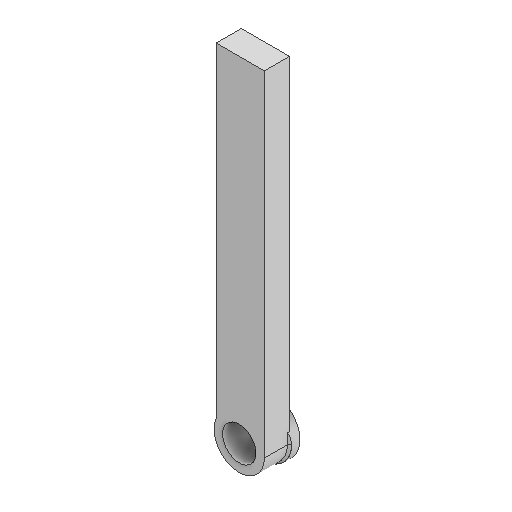
# Autodesk Inventor part: slide_clips_4mm
Saved by Autodesk Inventor 2023 (Build 270158000, 158)
## iProperties
Created: 2021-07-20
Part Number: slide_clips_4mm
Material: Generic
Document SubType Name: Modeling
Designer: CDT
Density: 1 g/cm^3
Appearance: Default
Author: CDT
Autodesk Inventor part; units mm, degrees
ref_plane "YZ Plane" through (0, 0, 0) normal (1, 0, 0) x (0, 1, 0)
ref_plane "XZ Plane" through (0, 0, 0) normal (0, 1, 0) x (-1, 0, 0)
ref_plane "XY Plane" through (0, 0, 0) normal (0, 0, 1) x (1, 0, 0)
sketch "Sketch1" plane through (0, 0, 0) normal (0, 0, 1) x (1, 0, 0)
  circle A0 centre (-24.0055, -25.7521) radius 3.25
  circle A1 centre (-24.0055, -25.7521) radius 2
  point P0 (0, 0)
  dimension "d0" = 6.5
  dimension "d1" = 4
  constraints: 2 centre point, 1 coincident
  measures "d0" diameter of A0
  measures "d1" diameter of A1
extrude "Extrusion1" add sketch "Sketch1" along normal blind 1
sketch "Sketch2" plane through (-24.0055, -25.7521, 1) normal (0, 0, 1) x (1, 0, 0)
  circle A0 centre (0, 0) radius 3
  circle A1 centre (0, 0) radius 2
  line L0 (0, 0) -> (-2.75, 0)
  line L1 (-2.75, 0) -> (-2.75, 40)
  line L2 (-2.75, 40) -> (0, 40)
  line L3 (0, 40) -> (0, 0)
  line L4 (0, 0) -> (3, 0)
  line L5 (3, 0) -> (3, 40)
  line L6 (3, 40) -> (0, 40)
  line L7 (0, 40) -> (0, 0)
  point P0 (24.0055, 25.7521)
  point P1 (-2.75, 1.199)
  point P2 (3, 0)
  point P3 (0, 40)
  dimension "d4" = 40
  dimension "d5" = 3
  dimension "d8" = 4
  dimension "d9" = 6
  constraints: 16 end point, 4 parallel, 2 centre point, 2 horizontal, 2 perpendicular, 1 coincident, 1 point on line
  measures "d4" distance of L0.end L1.end
  measures "d5" distance of L6.end L5.end
  measures "d8" diameter of A1
  measures "d9" diameter of A0
extrude "Extrusion2" add sketch "Sketch2" along normal blind 3 contours L4 A1 L3 A0 | A0 L1 L0 A1 L4 | A0 L3 L6 L5 | L3 A1 L0 L1 A0 | A0 L1 L2 L3
chamfer "Chamfer1" distance 0.245 angle 45 2 edges at (-24.6178, -28.689, 1) (-21.0055, -25.1271, 1)
body "Solid1"
